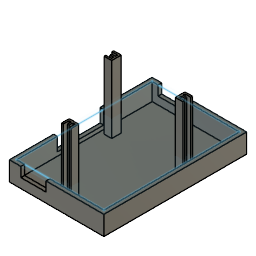
Deksel (Autodesk Fusion 360 design; units mm, degrees)
part number: 2026-04-23-15-00-40-917
Autodesk Fusion 360 part; units mm, degrees
sketch "Sketch1" plane through (0, 0, 0) normal (0, 0, 1) x (1, 0, 0)
  line L0 (0, 0) -> (49, 0)
  line L1 (49, 0) -> (49, 74)
  line L2 (49, 74) -> (0, 74)
  line L3 (0, 74) -> (0, 0)
  constraint horizontal L0
  constraint vertical L1
  constraint horizontal L2
  constraint vertical L3
  constraint coincident L0.start L3.end
extrude "Extrude1" add sketch "Sketch1" along normal blind 10
sketch "Sketch2" plane through (0, 0, 10) normal (0, 0, 1) x (-1, 0, 0)
  line L0 (0, -74) -> (0, 0)
  line L1 (0, 0) -> (-49, 0)
  line L2 (-49, 0) -> (-49, -74)
  line L3 (-49, -74) -> (0, -74)
  line L4 (-1.9, -72.1) -> (-47.1, -72.1)
  line L5 (-47.1, -72.1) -> (-47.1, -1.9)
  line L6 (-47.1, -1.9) -> (-1.9, -1.9)
  line L7 (-1.9, -1.9) -> (-1.9, -72.1)
  constraint horizontal L4
  constraint vertical L5
  constraint horizontal L6
  constraint vertical L7
extrude "Extrude2" cut sketch "Sketch2" against normal blind 9 contours L4 L5 L6 L7
sketch "Sketch3" plane through (0, 74, 0) normal (0, 1, 0) x (-1, 0, 0)
  line L0 (-49, 0) -> (0, 0)
  line L1 (0, 0) -> (0, 10)
  line L2 (0, 10) -> (-49, 10)
  line L3 (-49, 10) -> (-49, 0)
sketch "Sketch4" plane through (0, 74, 0) normal (0, 1, 0) x (-1, 0, 0)
  line L0 (-5, 5) -> (-19, 5)
  line L1 (-19, 5) -> (-19, 10)
  line L2 (-19, 10) -> (-5, 10)
  line L3 (-5, 10) -> (-5, 5)
  constraint horizontal L0
  constraint vertical L1
  constraint horizontal L2
  constraint vertical L3
extrude "Extrude3" cut sketch "Sketch4" against normal blind 6
sketch "Sketch5" plane through (0, 0, 0) normal (0, 1, 0) x (1, 0, 0)
sketch "Sketch6" plane through (0, 0, 0) normal (0, -1, 0) x (1, 0, 0)
  line L0 (0, 0) -> (49, 0)
  line L1 (49, 0) -> (49, 10)
  line L2 (49, 10) -> (0, 10)
  line L3 (0, 10) -> (0, 0)
  line L4 (6, 5) -> (19, 5)
  line L5 (19, 5) -> (19, 10)
  line L6 (19, 10) -> (6, 10)
  line L7 (6, 10) -> (6, 5)
  constraint horizontal L4
  constraint vertical L5
  constraint horizontal L6
  constraint vertical L7
  constraint coincident L2 L5.end
extrude "Extrude4" cut sketch "Sketch6" against normal blind 6 contours L2 L4 L5 L6 L7
sketch "Sketch7" plane through (0, 0, 0) normal (-1, 0, 0) x (0, -1, 0)
  line L0 (-74, 0) -> (0, 0)
  line L1 (0, 0) -> (0, 10)
  line L2 (0, 10) -> (-74, 10)
  line L3 (-74, 10) -> (-74, 0)
  line L4 (-23, 11) -> (-47, 11)
  line L5 (-47, 11) -> (-47, 3)
  line L6 (-47, 3) -> (-23, 3)
  line L7 (-23, 3) -> (-23, 11)
  constraint horizontal L4
  constraint vertical L5
  constraint horizontal L6
  constraint vertical L7
extrude "Extrude5" cut sketch "Sketch7" against normal blind 3 contours L2 L5 L6 L7
sketch "Sketch8" plane through (0, 0, 1) normal (0, 0, 1) x (-1, 0, 0)
  line L0 (-1.9, -1.9) -> (-47.1, -1.9)
  line L1 (-47.1, -1.9) -> (-47.1, -72.1)
  line L2 (-47.1, -72.1) -> (-1.9, -72.1)
  line L3 (-1.9, -72.1) -> (-1.9, -1.9)
  line L4 (-4.05, -50) -> (-8, -50)
  line L5 (-8, -50) -> (-8, -49.05)
  line L6 (-8, -49.05) -> (-4.05, -49.05)
  line L7 (-4.05, -49.05) -> (-4.05, -50)
  line L8 (-7, -49.05) -> (-8, -49.05)
  line L9 (-8, -49.05) -> (-8, -45.05)
  line L10 (-8, -45.05) -> (-7, -45.05)
  line L11 (-7, -45.05) -> (-7, -49.05)
  line L12 (-7, -45.05) -> (-4.05, -45.05)
  line L13 (-4.05, -45.05) -> (-4.05, -45.95)
  line L14 (-4.05, -45.95) -> (-7, -45.95)
  line L15 (-7, -45.95) -> (-7, -45.05)
  line L16 (-7, -47.05) -> (-5.05, -47.05)
  line L17 (-5.05, -47.05) -> (-5.05, -47.95)
  line L18 (-5.05, -47.95) -> (-7, -47.95)
  line L19 (-7, -47.95) -> (-7, -47.05)
  line L20 (-44.95, -50) -> (-41, -50)
  line L21 (-41, -50) -> (-41, -49.05)
  line L22 (-41, -49.05) -> (-44.95, -49.05)
  line L23 (-44.95, -49.05) -> (-44.95, -50)
  line L24 (-41, -49.05) -> (-42, -49.05)
  line L25 (-42, -49.05) -> (-42, -45)
  line L26 (-42, -45) -> (-41, -45)
  line L27 (-41, -45) -> (-41, -49.05)
  line L28 (-42, -47.95) -> (-43.95, -47.95)
  line L29 (-43.95, -47.95) -> (-43.95, -47.05)
  line L30 (-43.95, -47.05) -> (-42, -47.05)
  line L31 (-42, -47.05) -> (-42, -47.95)
  line L32 (-42, -45) -> (-44.95, -45)
  line L33 (-44.95, -45) -> (-44.95, -45.95)
  line L34 (-44.95, -45.95) -> (-42, -45.95)
  line L35 (-42, -45.95) -> (-42, -45)
  constraint horizontal L4
  constraint vertical L5
  constraint horizontal L6
  constraint vertical L7
  constraint horizontal L8
  constraint vertical L9
  constraint horizontal L10
  constraint vertical L11
  constraint coincident L6 L8.start
  constraint horizontal L12
  constraint vertical L13
  constraint horizontal L14
  constraint vertical L15
  constraint horizontal L16
  constraint vertical L17
  constraint horizontal L18
  constraint vertical L19
  constraint midpoint L11 L16.start
  constraint horizontal L20
  constraint vertical L21
  constraint horizontal L22
  constraint vertical L23
  constraint horizontal L24
  constraint vertical L25
  constraint horizontal L26
  constraint vertical L27
  constraint horizontal L28
  constraint vertical L29
  constraint horizontal L30
  constraint vertical L31
  constraint coincident L25 L28.start
  constraint horizontal L32
  constraint vertical L33
  constraint horizontal L34
  constraint vertical L35
extrude "Extrude6" add sketch "Sketch8" along normal blind 35 contours L4 L5 L6 L7 L8 | L6 L8 L9 L10 L11 L15 L19 | L11 L16 L17 L18 L19 | L11 L12 L13 L14 L15 | L20 L21 L22 L23 L24 | L22 L24 L25 L26 L27 L31 L35 | L25 L28 L29 L30 L31 | L25 L32 L33 L34 L35
sketch "Sketch9" plane through (0, 0, 0) normal (-1, 0, 0) x (0, -1, 0)
sketch "Sketch10" plane through (0, 0, 1) normal (0, 0, 1) x (-1, 0, 0)
  line L0 (-5.05, -47.95) -> (-7, -47.95)
  line L1 (-7, -47.95) -> (-7, -49.05)
  line L2 (-7, -49.05) -> (-4.05, -49.05)
  line L3 (-4.05, -49.05) -> (-4.05, -50)
  line L4 (-4.05, -50) -> (-8, -50)
  line L5 (-8, -50) -> (-8, -45.05)
  line L6 (-8, -45.05) -> (-4.05, -45.05)
  line L7 (-4.05, -45.05) -> (-4.05, -45.95)
  line L8 (-4.05, -45.95) -> (-7, -45.95)
  line L9 (-7, -45.95) -> (-7, -47.05)
  line L10 (-7, -47.05) -> (-5.05, -47.05)
  line L11 (-5.05, -47.05) -> (-5.05, -47.95)
  line L12 (-41, -45) -> (-41, -50)
  line L13 (-41, -50) -> (-44.95, -50)
  line L14 (-44.95, -50) -> (-44.95, -49.05)
  line L15 (-44.95, -49.05) -> (-42, -49.05)
  line L16 (-42, -49.05) -> (-42, -47.95)
  line L17 (-42, -47.95) -> (-43.95, -47.95)
  line L18 (-43.95, -47.95) -> (-43.95, -47.05)
  line L19 (-43.95, -47.05) -> (-42, -47.05)
  line L20 (-42, -47.05) -> (-42, -45.95)
  line L21 (-42, -45.95) -> (-44.95, -45.95)
  line L22 (-44.95, -45.95) -> (-44.95, -45)
  line L23 (-44.95, -45) -> (-41, -45)
  line L24 (-1.9, -1.9) -> (-47.1, -1.9)
  line L25 (-47.1, -1.9) -> (-47.1, -72.1)
  line L26 (-47.1, -72.1) -> (-1.9, -72.1)
  line L27 (-1.9, -72.1) -> (-1.9, -1.9)
  line L28 (-27.95, -4.05) -> (-27.05, -4.05)
  line L29 (-27.05, -4.05) -> (-27.05, -8)
  line L30 (-27.05, -8) -> (-27.95, -8)
  line L31 (-27.95, -8) -> (-27.95, -4.05)
  line L32 (-27.0625, -8) -> (-23.0375, -8)
  line L33 (-23.0375, -8) -> (-23.0375, -7)
  line L34 (-23.0375, -7) -> (-27.0625, -7)
  line L35 (-27.0625, -7) -> (-27.0625, -8)
  line L36 (-23.0375, -7) -> (-23.95, -7)
  line L37 (-23.95, -7) -> (-23.95, -4.05)
  line L38 (-23.95, -4.05) -> (-23.0375, -4.05)
  line L39 (-23.0375, -4.05) -> (-23.0375, -7)
  line L40 (-25.05, -7) -> (-25.95, -7)
  line L41 (-25.95, -7) -> (-25.95, -5.05)
  line L42 (-25.95, -5.05) -> (-25.05, -5.05)
  line L43 (-25.05, -5.05) -> (-25.05, -7)
  constraint horizontal L28
  constraint vertical L29
  constraint horizontal L30
  constraint vertical L31
  constraint horizontal L32
  constraint vertical L33
  constraint horizontal L34
  constraint vertical L35
  constraint horizontal L36
  constraint vertical L37
  constraint horizontal L38
  constraint vertical L39
  constraint horizontal L40
  constraint vertical L41
  constraint horizontal L42
  constraint vertical L43
  constraint midpoint L34 L40.start
extrude "Extrude7" add sketch "Sketch10" along normal blind 35 contours L28 L29 L30 L31 L34 L35 | L29 L32 L33 L34 L36 L40 | L29 L30 L32 L34 L35 | L34 L40 L41 L42 L43 | L34 L36 L37 L38 L39
